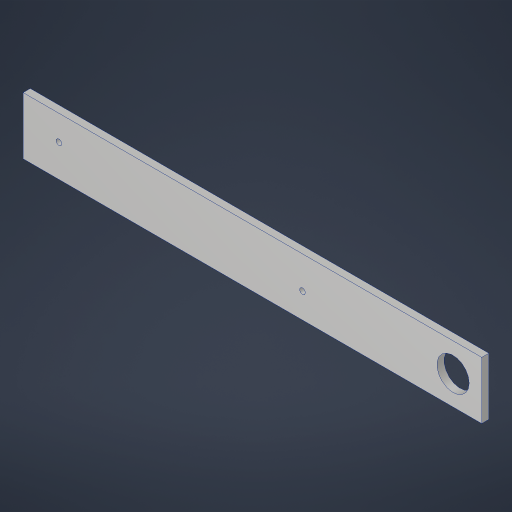
# Autodesk Inventor part: CL2-004
Saved by Autodesk Inventor 2023.4 (Build 274418000, 418)
## iProperties
Created: 2025-01-26
Part Number: CL2-004
Material: Aluminum 6061
Document SubType Name: Modeling
Designer: brand
Density: 2.7 g/cm^3
Appearance: Aluminum - Flat
Author: brand
Autodesk Inventor part; units mm, degrees
ref_plane "YZ Plane" through (0, 0, 0) normal (1, 0, 0) x (0, 1, 0)
ref_plane "XZ Plane" through (0, 0, 0) normal (0, 1, 0) x (-1, 0, 0)
ref_plane "XY Plane" through (0, 0, 0) normal (0, 0, 1) x (1, 0, 0)
sketch "Sketch1" plane through (0, 0, 0) normal (0, 0, 1) x (1, 0, 0)
  line L0 (-203.2, -25.4) -> (203.2, -25.4)
  line L1 (203.2, -25.4) -> (203.2, 25.4)
  line L2 (203.2, 25.4) -> (-203.2, 25.4)
  line L3 (-203.2, 25.4) -> (-203.2, -25.4)
  line L4 (-203.2, -25.4) -> (203.2, 25.4) construction
  line L5 (203.2, -25.4) -> (-203.2, 25.4) construction
  circle A0 centre (-171.45, 3.175) radius 14.2875 construction
  circle A1 centre (44.3566, -3.175) radius 14.2875 construction
  line L6 (-157.3708, 503.5787) -> (-157.3708, -106.0213) construction
  line L7 (-157.3708, -106.0213) -> (29.9542, -106.0213) construction
  line L8 (29.9542, -106.0213) -> (29.9542, 503.5787) construction
  line L9 (29.9542, 503.5787) -> (-157.3708, 503.5787) construction
  line L10 (-171.45, 3.175) -> (44.3566, -3.175) construction
  circle A2 centre (177.8, 0) radius 14.2875
  point P0 (0, 0)
  point P1 (-203.2, 0)
  point P2 (203.2, 0)
  dimension "d0" = 406.4
  dimension "d1" = 50.8
  dimension "d2" = 28.575
  dimension "d3" = 28.575
  dimension "d4" = 187.325
  dimension "d5" = 609.6
  dimension "d6" = 215.9
  dimension "d7" = 6.35
  dimension "d8" = 31.75
  dimension "d9" = 22.225
  dimension "d10" = 28.575
  dimension "d11" = 25.4
  constraints: 22 end point, 4 midpoint, 4 perpendicular, 3 centre point, 2 parallel, 1 horizontal, 1 horizontal alignment, 1 vertical
  measures "d0" distance of L2.end L1.end
  measures "d1" distance of L1.end L0.end
  measures "d2" diameter of A0
  measures "d3" diameter of A1
  measures "d4" distance of L6.end L7.end
  measures "d5" distance of L6.start L6.end
  measures "d6" distance of L10.start L10.end
  measures "d7" vertical distance of L10.end L10.start
  measures "d8" distance from line of L3 L10.start
  measures "d9" distance from line of L2 L10.start
  measures "d10" diameter of A2
  measures "d11" distance from line of L1 A2.centre
extrude "Extrusion1" add sketch "Sketch1" against normal blind 6.35
hole "Hole1" at (44.3566, -3.175, 0) at (-171.45, 3.175, 0) direction (0, 0, -1) diameter 5.1054 end through all clearance for "Flat Head Machine Screw (82)" size "#10" standard "Ansi Unified Screw Threads"
body "Solid1"
